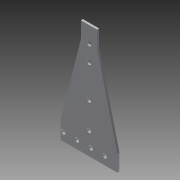
# Autodesk Inventor part: winch support
Saved by Autodesk Inventor 2013 (Build 170138000, 138)
## iProperties
Created: 2013-02-04
Part Number: winch support
Material: Aluminum 6061
Document SubType Name: Modeling
Designer: Arpan
Density: 2.71 g/cm^3
Mass: 85.6342 g
Surface Area: 218.201 cm^2
Volume: 31.5993 cm^3
Author: Arpan
Autodesk Inventor part; units mm, degrees
ref_plane "YZ Plane" through (0, 0, 0) normal (1, 0, 0) x (0, 1, 0)
ref_plane "XZ Plane" through (0, 0, 0) normal (0, 1, 0) x (-1, 0, 0)
ref_plane "XY Plane" through (0, 0, 0) normal (0, 0, 1) x (1, 0, 0)
sketch "Sketch1" plane through (0, 0, 0) normal (0, 0, 1) x (1, 0, 0)
  line L0 (0, 0) -> (-25.4, 0)
  line L1 (-25.4, 0) -> (-25.4, 177.8)
  line L2 (-25.4, 177.8) -> (0, 177.8)
  line L3 (0, 177.8) -> (0, 0)
  line L4 (-25.4, 0) -> (-57.15, 0)
  line L5 (0, 0) -> (31.75, 0)
  line L6 (31.75, 0) -> (31.75, 25.4)
  line L7 (31.75, 25.4) -> (0, 25.4)
  line L8 (-57.15, 0) -> (-57.15, 25.4)
  line L9 (-57.15, 25.4) -> (-25.4, 25.4)
  line L10 (31.75, 25.4) -> (28.575, 25.4)
  line L11 (-25.4, 177.8) -> (-25.4, 152.4)
  line L12 (0, 177.8) -> (0, 150.469)
  line L13 (0, 177.8) -> (0, 152.4)
  line L14 (-57.15, 25.4) -> (-25.4, 152.4)
  line L15 (0, 152.4) -> (31.75, 25.4)
  dimension "d0" = 177.8
  dimension "d3" = 25.4
  dimension "d4" = 31.75
  dimension "d5" = 31.75
  dimension "d6" = 25.4
  dimension "d7" = 3.175
  dimension "d16" = 25.4
  constraints: 32 end point, 6 perpendicular, 6 point on line, 3 equal length, 1 horizontal
  measures "d0" distance of L0.end L1.end
  measures "d3" distance of L0.start L0.end
  measures "d4" distance of L0.end L4.end
  measures "d5" distance of L0.start L5.end
  measures "d6" distance of L5.end L6.end
  measures "d7" distance of L6.end L10.end
  measures "d16" distance of L1.end L11.end
extrude "Extrusion1" add sketch "Sketch1" along normal blind 3.175
sketch "Sketch2" plane through (0, 0, 3.175) normal (0, 0, 1) x (1, 0, 0)
  line L0 (0, 177.8) -> (-25.4, 177.8) projected
  line L1 (-57.15, 25.4) -> (-57.15, 0) projected
  line L2 (-12.7, 177.8) -> (-12.7, 152.4)
  line L3 (-12.7, 152.4) -> (-12.7, 127)
  circle A0 centre (-12.7, 152.4) radius 3.3782
  circle A1 centre (-12.7, 127) radius 3.3782
  point P0 (0, 0)
  dimension "d10" = 25.4
  dimension "d11" = 25.4
  dimension "d12" = 6.7564
  dimension "d13" = 6.7564
  constraints: 4 end point, 2 centre point, 2 coincident, 2 equal length, 1 midpoint
  measures "d10" distance of L2.start L2.end
  measures "d11" distance of L2.end L3.end
  measures "d12" diameter of A0
  measures "d13" diameter of A1
extrude "Extrusion2" cut sketch "Sketch2" against normal blind 25.4
sketch "Sketch4" plane through (0, 0, 3.175) normal (0, 0, 1) x (1, 0, 0)
  circle A0 centre (11.6652, 12.7) radius 3.302 projected
  circle A1 centre (-9.8778, 12.7) radius 3.302 projected
  circle A2 centre (-52.9637, 12.7) radius 3.302 projected
  line L0 (74.422, 18.3438) -> (91.6421, 18.3438) projected
  circle A3 centre (-31.4207, 12.7) radius 3.302 projected
  point P0 (0, 0)
extrude "Extrusion3" cut sketch "Sketch4" against normal blind 25.4
sketch "Sketch5" plane through (0, 0, 3.175) normal (0, 0, 1) x (1, 0, 0)
  circle A0 centre (-12.7, 127) radius 3.3782 projected
  line L0 (-57.15, 25.4) -> (-57.15, 0) projected
  line L1 (-12.7, 127) -> (-12.7, 76.2)
  circle A1 centre (-12.7, 76.2) radius 3.3782
  point P0 (0, 0)
  dimension "d22" = 50.8
  dimension "d23" = 6.7564
  constraints: 2 end point, 1 centre point, 1 coincident, 1 parallel
  measures "d22" distance of L1.start L1.end
  measures "d23" diameter of A1
extrude "Extrusion4" cut sketch "Sketch5" against normal blind 25.4 contours A1
sketch "Sketch6" plane through (0, 0, 3.175) normal (0, 0, 1) x (1, 0, 0)
  circle A0 centre (-12.7, 76.2) radius 3.3782 projected
  line L0 (-57.15, 25.4) -> (-57.15, 0) projected
  line L1 (-12.7, 76.2) -> (-12.7, 34.925)
  circle A1 centre (-12.7, 34.925) radius 3.3782
  point P0 (0, 0)
  dimension "d26" = 41.275
  dimension "d27" = 6.7564
  constraints: 2 end point, 1 centre point, 1 coincident, 1 parallel
  measures "d26" distance of L1.start L1.end
  measures "d27" diameter of A1
extrude "Extrusion5" cut sketch "Sketch6" against normal blind 25.4 contours A1
body "Solid1"
